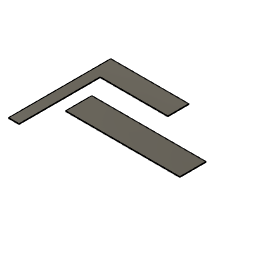
Bin stuff (Autodesk Fusion 360 design; units mm, degrees)
Autodesk Fusion 360 part; units mm, degrees
sketch "Sketch1" plane through (0, 0, 0) normal (0, 0, 1) x (1, 0, 0) in component "Bin lid"
  line L0 (0, 0) -> (380, 0)
  line L1 (380, 0) -> (380, 87)
  line L2 (380, 87) -> (0, 87)
  line L3 (0, 87) -> (0, 0)
  dimension "d1" = 380
  dimension "d2" = 87
  constraint horizontal L0
  constraint vertical L1
  constraint horizontal L2
  constraint vertical L3
  constraint coincident L0.start L3.end
  measures "d1" distance of L0.start L0.end
  measures "d2" distance of L0.start L2.end
extrude "Extrude1" add sketch "Sketch1" along normal blind 2 makes body 1 in component "Bin lid"
sketch "Sketch1 (2)" plane through (0, 0, 0) normal (0, 0, 1) x (1, 0, 0) in component "Bin guide"
  line L0 (-75, 225) -> (-75, -115)
  line L1 (185, 225) -> (-75, 225)
  line L2 (185, 155) -> (185, 225)
  line L3 (-40, -115) -> (-40, 155)
  line L4 (-40, 155) -> (185, 155)
  line L5 (-75, -115) -> (-40, -115)
extrude "Extrude1'" add sketch "Sketch1 (2)" along normal blind 2 separate body makes body 2 in component "Bin guide"
component "Bin lid" placed x (1, 0, 0) y (0, 1, 0) z (0, 0, 1) at (0, 0, 0)
component "Bin guide" placed x (1, 0, 0) y (0, 1, 0) z (0, 0, 1) at (0, 0, 0)
